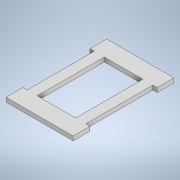
# Autodesk Inventor part: TopHolderV1
Saved by Autodesk Inventor 2020 (Build 240168000, 168)
## iProperties
Created: 2020-06-07
Part Number: TopHolderV1
Material: Generic
Document SubType Name: Modeling
Designer: Kitte_x
Density: 1 g/cm^3
Appearance: Default
Author: Kitte_x
Autodesk Inventor part; units mm, degrees
ref_plane "YZ Plane" through (0, 0, 0) normal (1, 0, 0) x (0, 1, 0)
ref_plane "XZ Plane" through (0, 0, 0) normal (0, 1, 0) x (-1, 0, 0)
ref_plane "XY Plane" through (0, 0, 0) normal (0, 0, 1) x (1, 0, 0)
sketch "Sketch1" plane through (0, 0, 0) normal (0, 1, 0) x (-1, 0, 0)
  line L0 (50, 75) -> (-50, 75)
  line L1 (-50, -75) -> (50, -75)
  line L2 (50, 50) -> (43.65, 50)
  line L3 (43.65, 50) -> (43.65, -50)
  line L4 (43.65, -50) -> (50, -50)
  line L5 (-50, 50) -> (-43.65, 50)
  line L6 (-43.65, 50) -> (-43.65, -50)
  line L7 (-43.65, -50) -> (-50, -50)
  line L8 (50, -75) -> (50, -50)
  line L9 (50, 50) -> (50, 75)
  line L10 (-50, 75) -> (-50, 50)
  line L11 (-50, -50) -> (-50, -75)
  line L12 (28.65, 50) -> (-28.65, 50)
  line L13 (-28.65, 50) -> (-28.65, -50)
  line L14 (-28.65, -50) -> (28.65, -50)
  line L15 (28.65, -50) -> (28.65, 50)
  point P0 (0, 0)
  point P1 (50, 0)
  point P2 (0, -75)
  point P3 (43.65, 0)
  point P4 (28.65, 0)
  point P5 (0, -50)
  point P6 (0, 50)
  point P7 (46.825, 50)
  dimension "d1" = 150
  dimension "d5" = 25
  dimension "d6" = 25
  dimension "d7" = 6.35
  dimension "d8" = 6.35
  dimension "d9" = 100
  dimension "d10" = 100
  dimension "d11" = 6.35
  dimension "d12" = 15
  constraints: 32 end point, 11 perpendicular, 6 midpoint, 4 horizontal alignment, 4 point on line, 3 horizontal, 2 parallel, 2 vertical alignment
  measures "d1" distance of L0.end L1.start
  measures "d5" distance between parallel lines of L1 L7
  measures "d6" distance between parallel lines of L0 L5
  measures "d7" distance between parallel lines of L6 L10
  measures "d8" distance between parallel lines of L9 L3
  measures "d9" distance between parallel lines of L11 L8
  measures "d10" distance of L0.start L0.end
  measures "d11" distance between parallel lines of L8 L3
  measures "d12" distance between parallel lines of L3 L15
extrude "Extrusion1" add sketch "Sketch1" along normal blind 6.35
body "Solid1"
